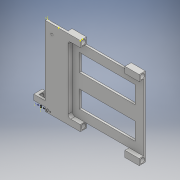
# Autodesk Inventor part: mtv_frontHolder(4_30)
Saved by Autodesk Inventor 2018 (Build 220112000, 112)
## iProperties
Created: 2019-04-30
Part Number: mtv_frontHolder(4_30)
Material: Generic
Document SubType Name: Modeling
Designer: Aditya Kendre
Density: 1 g/cm^3
Appearance: Default
Author: Aditya Kendre
## iProperties of the stored document mtv_frontHolder(4_30)_3DPrint.ipt
Created: 2019-04-30
Part Number: mtv_frontHolder(4_30)_3DPrint
Material: Generic
Document SubType Name: Modeling
Designer: Aditya Kendre
Density: 1 g/cm^3
Appearance: Default
Author: Aditya Kendre
Autodesk Inventor part; units mm, degrees
ref_plane "YZ Plane" through (0, 0, 0) normal (1, 0, 0) x (0, 1, 0)
ref_plane "XZ Plane" through (0, 0, 0) normal (0, 1, 0) x (-1, 0, 0)
ref_plane "XY Plane" through (0, 0, 0) normal (0, 0, 1) x (1, 0, 0)
sketch "Sketch1" plane through (0, 0, 0) normal (1, 0, 0) x (0, 1, 0)
  line L0 (0, 0) -> (8.763, 0)
  line L1 (8.763, 0) -> (8.763, -5.5118)
  line L2 (8.763, -5.5118) -> (0, -5.5118)
  line L3 (0, -5.5118) -> (0, 0)
  line L4 (1.5875, -3.9243) -> (7.1755, -3.9243)
  line L5 (7.1755, -3.9243) -> (7.1755, -1.5875)
  line L6 (7.1755, -1.5875) -> (1.5875, -1.5875)
  line L7 (1.5875, -1.5875) -> (1.5875, -3.9243)
  line L8 (1.5875, -3.9243) -> (7.1755, -1.5875) construction
  line L9 (7.1755, -3.9243) -> (1.5875, -1.5875) construction
  line L10 (0, -105.512) -> (8.763, -105.512)
  line L11 (8.763, -105.512) -> (8.763, -111.0238)
  line L12 (8.763, -111.0238) -> (0, -111.0238)
  line L13 (0, -111.0238) -> (0, -105.512)
  line L14 (1.5875, -109.4363) -> (7.1755, -109.4363)
  line L15 (7.1755, -109.4363) -> (7.1755, -107.0995)
  line L16 (7.1755, -107.0995) -> (1.5875, -107.0995)
  line L17 (1.5875, -107.0995) -> (1.5875, -109.4363)
  line L18 (1.5875, -109.4363) -> (7.1755, -107.0995) construction
  line L19 (7.1755, -109.4363) -> (1.5875, -107.0995) construction
  point P0 (4.3815, -2.7559)
  point P1 (4.3815, -108.2679)
  dimension "d0" = 8.763
  dimension "d1" = 5.5118
  dimension "d2" = 5.588
  dimension "d3" = 2.3368
  dimension "d4" = 8.763
  dimension "d5" = 5.5118
  dimension "d6" = 5.588
  dimension "d7" = 2.3368
  constraints: 40 end point, 8 parallel, 4 horizontal, 4 midpoint, 4 perpendicular, 1 point on line
  measures "d0" distance of L1.end L2.end
  measures "d1" distance of L0.end L1.end
  measures "d2" distance of L6.end L5.end
  measures "d3" distance of L5.end L4.end
  measures "d4" distance of L11.end L12.end
  measures "d5" distance of L10.end L11.end
  measures "d6" distance of L16.end L15.end
  measures "d7" distance of L15.end L14.end
extrude "Extrusion1" add sketch "Sketch1" against normal blind 30
sketch "Sketch2" plane through (-30, 0, 0) normal (-1, 0, 0) x (0, 0, 1)
  line L0 (0, 0) -> (0, 8.763) projected
  line L1 (-111.0238, 0) -> (0, 0)
  line L2 (0, 0) -> (0, 8.763)
  line L3 (0, 8.763) -> (-111.0238, 8.763)
  line L4 (-111.0238, 8.763) -> (-111.0238, 0)
  constraints: 8 end point, 2 parallel, 1 horizontal, 1 perpendicular
extrude "Extrusion2" add sketch "Sketch2" along normal blind 0.25
fillet "Fillet1" radius 5 2 edges at (-30, 4.3815, -5.5118) (-30, 4.3815, -105.512)
sketch "Sketch3" plane through (-30.25, 0, 0) normal (-1, 0, 0) x (0, 0, 1)
  point P0 (0, 0)
sketch "Sketch4" plane through (-30.25, 0, 0) normal (-1, 0, 0) x (0, 0, 1)
  line L0 (-111.0238, 8.763) -> (-111.0238, 0) projected
  line L1 (0, 0) -> (-111.0238, 0)
  line L2 (-111.0238, 0) -> (-111.0238, 3)
  line L3 (-111.0238, 3) -> (0, 3)
  line L4 (0, 3) -> (0, 0)
  dimension "d13" = 3
  constraints: 8 end point, 2 parallel, 1 horizontal, 1 perpendicular, 1 point on line
  measures "d13" distance of L1.end L2.end
extrude "Extrusion3" add sketch "Sketch4" along normal blind 18.97
sketch "Sketch5" plane through (-30.25, 3, 0) normal (0, 1, 0) x (1, 0, 0)
  line L0 (0, 0) -> (0, 111.0238) construction
  line L1 (0, 0) -> (-9.485, 0) construction
  line L2 (-9.485, 0) -> (-9.485, 6.985) construction
  line L3 (-9.485, 6.985) -> (0, 6.985) construction
  line L4 (0, 6.985) -> (0, 0) construction
  circle A0 centre (-9.485, 6.985) radius 1.5875
  point P0 (30.25, 0)
  dimension "d16" = 9.485
  dimension "d17" = 6.985
  dimension "d18" = 3.175
  constraints: 8 end point, 2 parallel, 1 centre point, 1 coincident, 1 horizontal, 1 perpendicular
  measures "d16" distance of L2.end L3.end
  measures "d17" distance of L1.end L2.end
  measures "d18" diameter of A0
extrude "Extrusion4" cut sketch "Sketch5" against normal blind 5
sketch "Sketch6" plane through (-30.25, 3, 0) normal (0, 1, 0) x (1, 0, 0)
  line L0 (30.25, 111.0238) -> (-18.97, 111.0238) construction
  line L1 (-28.07, 111.0238) -> (-28.07, 111.0238) construction
  line L2 (-28.07, 111.0238) -> (-28.07, 111.0238) construction
  line L3 (-28.07, 111.0238) -> (-28.07, 111.0238) construction
  line L4 (-28.07, 111.0238) -> (-28.07, 111.0238) construction
  line L5 (-28.07, 111.0238) -> (-28.07, 111.0238) construction
  line L6 (-28.07, 118.8238) -> (-28.07, 111.0238) construction
  line L7 (-28.07, 111.0238) -> (-37.17, 111.0238) construction
  line L8 (-37.17, 111.0238) -> (-37.17, 114.8988) construction
  line L9 (-28.07, 111.0238) -> (-28.07, 111.0238) construction
  line L10 (-28.07, 111.0238) -> (-28.07, 111.0238) construction
  line L11 (-28.07, 111.0238) -> (-28.07, 111.0238) construction
  line L12 (-28.07, 111.0238) -> (-28.07, 111.0238) construction
  line L13 (-28.07, 111.0238) -> (-28.07, 111.0238) construction
  line L14 (-28.07, 111.0238) -> (-28.07, 111.0238)
  line L15 (-28.07, 111.0238) -> (-28.07, 111.0238)
  line L16 (-28.07, 111.0238) -> (-28.07, 111.0238)
  line L17 (-28.07, 111.0238) -> (-28.07, 111.0238)
  point P0 (30.25, 0)
  dimension "d21" = 0
  dimension "d22" = 0
  dimension "d23" = 0
  dimension "d26" = 0
  dimension "d27" = 0
  constraints: 34 end point, 6 collinear, 4 horizontal, 4 perpendicular, 1 parallel, 1 point on line, 1 vertical
  measures "d21" distance of L3.end L2.end
  measures "d22" distance of L1.end L2.end
  measures "d23" distance of L2.end L5.end
  measures "d26" distance of L11.end L10.end
  measures "d27" distance of L9.start L10.end
sketch "Sketch7" plane through (-30.25, 3, 0) normal (0, 1, 0) x (1, 0, 0)
  line L0 (-18.97, 0) -> (-18.97, 111.0238) projected
  line L1 (-18.97, 111.0238) -> (-27.97, 111.0238)
  line L2 (-27.97, 111.0238) -> (-27.97, 103.2738)
  line L3 (-27.97, 103.2738) -> (-18.97, 103.2738)
  line L4 (-18.97, 103.2738) -> (-18.97, 111.0238)
  point P0 (30.25, 0)
  dimension "d28" = 9
  dimension "d29" = 7.75
  constraints: 8 end point, 2 parallel, 1 horizontal, 1 perpendicular
  measures "d28" distance of L3.end L2.end
  measures "d29" distance of L2.end L1.end
extrude "Extrusion5" add sketch "Sketch7" against normal blind 3
sketch "Sketch8" plane through (-30.25, 3, 0) normal (0, 1, 0) x (1, 0, 0)
  line L0 (-27.97, 111.0238) -> (-27.97, 103.2738) projected
  line L1 (-27.97, 111.0238) -> (-31.97, 111.0238)
  line L2 (-31.97, 111.0238) -> (-31.97, 103.2738)
  line L3 (-31.97, 103.2738) -> (-27.97, 103.2738)
  line L4 (-27.97, 103.2738) -> (-27.97, 111.0238)
  point P0 (30.25, 0)
  dimension "d32" = 4
  constraints: 8 end point, 2 parallel, 1 horizontal, 1 perpendicular
  measures "d32" distance of L3.end L2.end
extrude "Extrusion6" add sketch "Sketch8" along normal blind 8 and the other way blind 3
sketch "Sketch9" plane through (0, 0, -5.5118) normal (0, -1, 0) x (1, 0, 0)
  point P0 (0, 5.5118)
sketch "Sketch10" plane through (-62.22, 0, -103.2738) normal (-1, 0, 0) x (0, 0, 1)
  line L0 (-7.75, 0) -> (-2.2382, 0) construction
  line L1 (0, 3) -> (0, 11) construction
  line L2 (-7.75, 0) -> (0, 0) construction
  line L3 (0, 0) -> (0, 3) construction
  line L4 (0, 3) -> (-7.75, 3) construction
  line L5 (-7.75, 3) -> (-7.75, 0) construction
  line L6 (103.2738, 3) -> (0, 3) construction
  line L7 (-7.75, 8.763) -> (-7.75, 3) construction
  line L8 (0, 3) -> (-7.75, 3) construction
  line L9 (-7.75, 3) -> (-7.75, 6.875) construction
  line L10 (-7.75, 6.875) -> (0, 6.875) construction
  line L11 (0, 6.875) -> (0, 3) construction
  circle A0 centre (-3.875, 6.875) radius 3.1
  point P0 (103.2738, 0)
  dimension "d37" = 3.875
  dimension "d38" = 6.2
  constraints: 16 end point, 4 parallel, 2 horizontal, 2 perpendicular, 1 centre point, 1 midpoint, 1 point on line
  measures "d37" distance of L8.end L9.end
  measures "d38" diameter of A0
extrude "Extrusion7" cut sketch "Sketch10" against normal blind 5
sketch "Sketch11" plane through (0, 8.763, 0) normal (0, 1, 0) x (1, 0, 0)
  line L0 (-30.25, 111.0238) -> (-30.25, 0) projected
  line L1 (0, 0) -> (-30.25, 0) projected
  line L2 (-30.25, 111.0238) -> (-20.25, 111.0238)
  line L3 (-20.25, 111.0238) -> (-20.25, 0)
  line L4 (-20.25, 0) -> (-30.25, 0)
  line L5 (-30.25, 0) -> (-30.25, 111.0238)
  dimension "d41" = 10
  constraints: 8 end point, 2 parallel, 1 horizontal, 1 perpendicular, 1 point on line
  measures "d41" distance of L3.end L4.end
extrude "Extrusion8" cut sketch "Sketch11" against normal blind 10
sketch "Sketch12" plane through (-30.25, 0, 0) normal (1, 0, 0) x (0, 0, -1)
  line L0 (111.0238, 3) -> (111.0238, 0) projected
  line L1 (0, 0) -> (111.0238, 0)
  line L2 (111.0238, 0) -> (111.0238, 3)
  line L3 (111.0238, 3) -> (0, 3)
  line L4 (0, 3) -> (0, 0)
  constraints: 8 end point, 2 parallel, 1 horizontal, 1 perpendicular
extrude "Extrusion9" add sketch "Sketch12" along normal blind 13
sketch "Sketch13" plane through (0, 8.763, 0) normal (0, 1, 0) x (1, 0, 0)
  line L0 (-20.25, 5.5118) -> (-20.25, 0) projected
  line L1 (-62.22, 111.0238) -> (0, 111.0238) projected
  line L2 (-20.25, 0) -> (-17.25, 0)
  line L3 (-17.25, 0) -> (-17.25, 111.0238)
  line L4 (-17.25, 111.0238) -> (-20.25, 111.0238)
  line L5 (-20.25, 111.0238) -> (-20.25, 0)
  point P0 (0, 0)
  dimension "d46" = 3
  constraints: 8 end point, 2 parallel, 1 horizontal, 1 perpendicular, 1 point on line
  measures "d46" distance of L4.end L3.end
extrude "Extrusion10" add sketch "Sketch13" against normal blind 8.75
sketch "Sketch14" plane through (-49.22, 3, 0) normal (0, 1, 0) x (1, 0, 0)
  line L0 (-9, 111.0238) -> (28.97, 111.0238) construction
  line L1 (0, 0) -> (0, 0) construction
  line L2 (0, 0) -> (0, 111.0238) construction
  line L3 (0, 111.0238) -> (0, 111.0238) construction
  line L4 (0, 111.0238) -> (0, 0) construction
  point P0 (49.22, 0)
  dimension "d49" = 0
  constraints: 8 end point, 2 equal length, 1 horizontal, 1 perpendicular, 1 point on line
  measures "d49" distance of L3.end L2.end
sketch "Sketch15" plane through (-49.22, 3, 0) normal (0, 1, 0) x (1, 0, 0)
  line L0 (0, 107.1488) -> (28.97, 107.1488) construction
  line L1 (28.97, 111.0238) -> (28.97, 0) construction
  point P0 (49.22, 0)
  constraints: 2 end point, 1 horizontal, 1 point on line
sketch "Sketch16" plane through (-20.25, 8.763, -111.0238) normal (-1, 0, 0) x (0, 0, 1)
  line L0 (0, 0) -> (111.0238, 0) construction
  line L1 (0, 0) -> (7.7501, 0) construction
  line L2 (0, -5.763) -> (111.0238, -5.763) construction
  line L3 (0, 0) -> (7.7501, 0) construction
  line L4 (7.7501, 0) -> (7.7501, -5.763) construction
  line L5 (7.7501, -5.763) -> (0, -5.763) construction
  line L6 (0, -5.763) -> (0, 0) construction
  line L7 (0, -5.763) -> (4.375, -5.763) construction
  line L8 (4.375, -5.763) -> (4.375, -1.388) construction
  line L9 (4.375, -1.388) -> (0, -1.388) construction
  line L10 (0, -1.388) -> (0, -5.763) construction
  circle A0 centre (4.375, -1.388) radius 1.5
  point P0 (111.0238, -8.763)
  dimension "d52" = 4.375
  dimension "d53" = 4.375
  dimension "d54" = 3
  constraints: 18 end point, 4 parallel, 2 horizontal, 2 perpendicular, 2 point on line, 1 centre point, 1 coincident
  measures "d52" distance of L9.end L8.end
  measures "d53" distance of L8.end L7.end
  measures "d54" diameter of A0
extrude "Extrusion11" add sketch "Sketch16" along normal blind 2
sketch "Sketch17" plane through (-49.22, 3, 0) normal (0, 1, 0) x (1, 0, 0)
  circle A0 centre (9.485, 6.985) radius 1.5875 construction
  line L0 (0, 0) -> (0, 103.2738) construction
  line L1 (9.485, 6.985) -> (0, 6.985) construction
  line L2 (0, 6.985) -> (0, 0) construction
  line L3 (0, 0) -> (9.485, 0) construction
  line L4 (9.485, 0) -> (9.485, 6.985) construction
  line L5 (31.97, 5.5118) -> (31.97, 105.512) construction
  line L6 (31.97, 5.5118) -> (0, 5.5118) construction
  line L7 (0, 5.5118) -> (0, 12.4968) construction
  line L8 (0, 12.4968) -> (31.97, 12.4968) construction
  line L9 (31.97, 12.4968) -> (31.97, 5.5118) construction
  circle A1 centre (9.485, 12.4968) radius 1.5
  circle A2 centre (9.485, 6.985) radius 1.4732
  circle A3 centre (9.485, 6.985) radius 2.1184
  point P0 (49.22, 0)
  dimension "d57" = 9.485
  dimension "d58" = 6.985
  dimension "d59" = 6.985
  dimension "d60" = 3
  constraints: 16 end point, 4 parallel, 3 centre point, 3 coincident, 2 horizontal, 2 perpendicular, 2 point on line
  measures "d57" distance of L0.start L3.end
  measures "d58" distance of L0.start L1.end
  measures "d59" distance of L6.end L7.end
  measures "d60" diameter of A1
extrude "Extrusion12" cut sketch "Sketch17" against normal blind 3 contours A1
sketch "Sketch18" plane through (-49.22, 3, 0) normal (0, 1, 0) x (1, 0, 0)
  circle A0 centre (9.485, 6.985) radius 1.5875 projected
  circle A1 centre (9.485, 6.985) radius 2.2024
  point P0 (49.22, 0)
  constraints: 1 centre point, 1 coincident
extrude "Extrusion13" add sketch "Sketch18" against normal blind 3 contours A0 | A1
sketch "Sketch19" plane through (-49.22, 3, 0) normal (0, 1, 0) x (1, 0, 0)
  line L0 (49.22, 5.5118) -> (31.97, 5.5118) construction
  line L1 (31.97, 5.5118) -> (0, 5.5118) construction
  line L2 (31.97, 105.5118) -> (31.97, 5.5118) construction
  line L3 (0, 103.2738) -> (0, 0) construction
  line L4 (0, 103.2738) -> (-13.792, 103.2738) construction
  line L5 (-13.792, 103.2738) -> (-13.792, 112.9328) construction
  line L6 (-13.792, 112.9328) -> (0, 112.9328) construction
  line L7 (0, 112.9328) -> (0, 103.2738) construction
  line L8 (-9, 103.2738) -> (0, 103.2738) projected
  line L9 (0, 103.2738) -> (-14.6847, 103.2738)
  line L10 (-14.6847, 103.2738) -> (-14.6847, 119.5752)
  line L11 (-14.6847, 119.5752) -> (0, 119.5752)
  line L12 (0, 119.5752) -> (0, 103.2738)
  point P0 (49.22, 0)
  constraints: 20 end point, 4 parallel, 3 horizontal, 2 perpendicular
extrude "Extrusion14" cut sketch "Sketch19" along normal mid plane 30
sketch "Sketch20" plane through (-49.22, 3, 0) normal (0, 1, 0) x (1, 0, 0)
  line L0 (31.97, 5.5118) -> (31.97, 105.512) construction
  line L1 (0, 0) -> (0, 111.0238) construction
  line L2 (31.97, 5.5118) -> (0, 5.5118) construction
  line L3 (0, 5.5118) -> (0, 105.5118) construction
  line L4 (0, 105.5118) -> (31.97, 105.5118) construction
  line L5 (31.97, 105.5118) -> (31.97, 5.5118) construction
  line L6 (0, 105.5118) -> (-12.042, 105.5118)
  line L7 (-12.042, 105.5118) -> (-12.042, 97.7618)
  line L8 (-12.042, 97.7618) -> (0, 97.7618)
  line L9 (0, 97.7618) -> (0, 105.5118)
  point P0 (49.22, 0)
  dimension "d68" = 100
  dimension "d69" = 12.042
  dimension "d70" = 7.75
  constraints: 16 end point, 4 parallel, 2 horizontal, 2 perpendicular, 1 point on line
  measures "d68" distance of L2.end L3.end
  measures "d69" distance of L8.end L7.end
  measures "d70" distance of L7.end L6.end
extrude "Extrusion15" add sketch "Sketch20" against normal blind 3
sketch "Sketch21" plane through (-49.22, 3, 0) normal (0, 1, 0) x (1, 0, 0)
  line L0 (-12.042, 97.7618) -> (0, 97.7618) projected
  line L1 (-12.042, 97.7618) -> (-16.042, 97.7618)
  line L2 (-16.042, 97.7618) -> (-16.042, 105.5118)
  line L3 (-16.042, 105.5118) -> (-12.042, 105.5118)
  line L4 (-12.042, 105.5118) -> (-12.042, 97.7618)
  point P0 (49.22, 0)
  dimension "d73" = 4
  constraints: 8 end point, 2 parallel, 1 horizontal, 1 perpendicular
  measures "d73" distance of L2.end L3.end
extrude "Extrusion16" add sketch "Sketch21" along normal blind 9 and the other way blind 3
sketch "Sketch22" plane through (-65.262, 0, -97.7618) normal (-1, 0, 0) x (0, 0, 1)
  line L0 (-13.262, 3) -> (97.7618, 3) construction
  line L1 (0, 3) -> (-7.75, 3) construction
  line L2 (-7.75, 0) -> (-7.75, 3) construction
  line L3 (-7.75, 3) -> (-3.875, 3) construction
  line L4 (-3.875, 3) -> (-3.875, 6.875) construction
  line L5 (-3.875, 6.875) -> (-7.75, 6.875) construction
  line L6 (-7.75, 6.875) -> (-7.75, 3) construction
  circle A0 centre (-3.875, 6.875) radius 3.1
  point P0 (97.7618, 0)
  dimension "d78" = 7.75
  dimension "d79" = 3.875
  dimension "d80" = 3.875
  dimension "d81" = 6.2
  constraints: 10 end point, 2 parallel, 2 point on line, 1 centre point, 1 coincident, 1 horizontal, 1 perpendicular
  measures "d78" distance of L1.start L1.end
  measures "d79" distance of L5.end L4.end
  measures "d80" distance of L4.end L3.end
  measures "d81" diameter of A0
extrude "Extrusion17" cut sketch "Sketch22" against normal blind 4
sketch "Sketch23" plane through (-49.22, 3, 0) normal (0, 1, 0) x (1, 0, 0)
  point P0 (49.22, 0)
sketch "Sketch24" plane through (-20.25, 3, -111.0238) normal (-1, 0, 0) x (0, 0, 1)
  line L0 (0, 5.763) -> (3.8063, 5.763) construction
  line L1 (0, 0) -> (111.0238, 0) construction
  line L2 (0, 5.763) -> (5.512, 5.763) construction
  line L3 (5.512, 5.763) -> (5.512, 0) construction
  line L4 (5.512, 0) -> (0, 0) construction
  line L5 (0, 0) -> (0, 5.763) construction
  line L6 (5.512, 0) -> (9.887, 0) construction
  line L7 (9.887, 0) -> (9.887, 4.375) construction
  line L8 (9.887, 4.375) -> (5.512, 4.375) construction
  line L9 (5.512, 4.375) -> (5.512, 0) construction
  circle A0 centre (9.887, 4.375) radius 1.5
  point P0 (111.0238, -3)
  dimension "d84" = 5.512
  dimension "d85" = 4.375
  dimension "d86" = 4.375
  dimension "d87" = 3
  constraints: 16 end point, 4 parallel, 2 horizontal, 2 perpendicular, 1 centre point, 1 coincident, 1 point on line
  measures "d84" distance of L3.end L4.end
  measures "d85" distance of L8.end L7.end
  measures "d86" distance of L7.end L6.end
  measures "d87" diameter of A0
extrude "Extrusion18" add sketch "Sketch24" along normal blind 3
sketch "Sketch25" plane through (-22.25, 7.375, -106.6488) normal (-1, 0, 0) x (0, 0, 1)
  circle A0 centre (0, 0) radius 1.5
  point P0 (106.6488, -7.375)
  constraints: 1 centre point
extrude "Extrusion19" cut sketch "Sketch25" against normal blind 2
sketch "Sketch26" plane through (0, 0, 0) normal (1, 0, 0) x (0, 0, -1)
  line L0 (0, 0) -> (0, 8.763) projected
  line L1 (0, 8.763) -> (8.763, 8.763)
  line L2 (8.763, 8.763) -> (8.763, 0)
  line L3 (8.763, 0) -> (0, 0)
  line L4 (0, 0) -> (0, 8.763)
  line L5 (105.512, 8.763) -> (111.0238, 8.763) projected
  line L6 (5.5118, 0) -> (105.512, 0) projected
  line L7 (111.0238, 8.763) -> (102.2608, 8.763)
  line L8 (102.2608, 8.763) -> (102.2608, 0)
  line L9 (102.2608, 0) -> (111.0238, 0)
  line L10 (111.0238, 0) -> (111.0238, 8.763)
  dimension "d92" = 8.763
  dimension "d93" = 8.763
  constraints: 16 end point, 4 parallel, 2 horizontal, 2 perpendicular, 1 point on line
  measures "d92" distance of L2.end L3.end
  measures "d93" distance of L9.end L8.end
extrude "Extrusion20" add sketch "Sketch26" against normal blind 20.25
sketch "Sketch27" plane through (-49.22, 3, 0) normal (0, 1, 0) x (1, 0, 0)
  point P0 (49.22, 0)
sketch "Sketch28" plane through (0, 0, 0) normal (1, 0, 0) x (0, 0, -1)
  line L0 (0, 8.763) -> (8.763, 8.763) construction
  line L1 (0, 8.763) -> (8.763, 0) construction
  line L2 (8.763, 0) -> (8.763, 8.763) construction
  line L3 (97.7618, 0) -> (0, 0) construction
  line L4 (8.763, 8.763) -> (0, 0) construction
  line L5 (111.0238, 8.763) -> (102.2608, 8.763) construction
  line L6 (111.0238, 8.763) -> (111.0238, 0) construction
  line L7 (102.2608, 8.763) -> (111.0238, 0) construction
  line L8 (111.0238, 0) -> (111.0238, 8.763) construction
  line L9 (111.0238, 8.763) -> (102.2608, 0) construction
  circle A0 centre (106.6423, 4.3815) radius 3.25
  circle A1 centre (4.3815, 4.3815) radius 3.25
  dimension "d96" = 6.5
  dimension "d97" = 6.5
  constraints: 12 end point, 2 centre point, 2 midpoint, 2 perpendicular, 1 collinear, 1 vertical
  measures "d96" diameter of A0
  measures "d97" diameter of A1
extrude "Extrusion21" cut sketch "Sketch28" against normal blind 17.25
fillet "Fillet2" radius 4 2 edges at (-17.25, 4.3815, -8.763) (-17.25, 4.3815, -102.2608)
sketch "Sketch29" plane through (-17.25, 0, 0) normal (1, 0, 0) x (0, 0, -1)
  line L0 (8.763, 0) -> (8.763, 8.763) projected
  line L1 (102.2608, 0) -> (102.2608, 8.763) projected
  line L2 (8.763, 8.763) -> (102.2608, 8.763)
  line L3 (102.2608, 8.763) -> (102.2608, 6.013)
  line L4 (102.2608, 6.013) -> (8.763, 6.013)
  line L5 (8.763, 6.013) -> (8.763, 8.763)
  point P0 (0, 0)
  dimension "d101" = 2.75
  constraints: 8 end point, 2 parallel, 1 horizontal, 1 perpendicular, 1 point on line
  measures "d101" distance of L2.end L3.end
extrude "Extrusion22" add sketch "Sketch29" along normal blind 100
sketch "Sketch30" plane through (-20.25, 8.763, -111.0238) normal (0, 1, 0) x (1, 0, 0)
  line L0 (103, -102.2608) -> (103, -8.763) construction
  line L1 (103, -102.2608) -> (3, -102.2608) construction
  line L2 (3, -102.2608) -> (3, -8.763) construction
  line L3 (3, -8.763) -> (103, -8.763) construction
  line L4 (103, -8.763) -> (103, -102.2608) construction
  line L5 (3, -98.2608) -> (3, -12.763) construction
  line L6 (3, -55.5119) -> (103, -55.5119) construction
  line L7 (3, -55.5119) -> (101.425, -55.5119) construction
  line L8 (101.425, -55.5119) -> (101.425, -99.9619) construction
  line L9 (101.425, -99.9619) -> (3, -99.9619) construction
  line L10 (3, -99.9619) -> (3, -55.5119) construction
  line L11 (3, -55.5119) -> (101.425, -55.5119) construction
  line L12 (101.425, -55.5119) -> (101.425, -11.0619) construction
  line L13 (101.425, -11.0619) -> (3, -11.0619) construction
  line L14 (3, -11.0619) -> (3, -55.5119) construction
  line L15 (101.425, -55.5119) -> (91.425, -55.5119) construction
  line L16 (91.425, -55.5119) -> (91.425, -11.0619) construction
  line L17 (91.425, -11.0619) -> (91.425, -21.0619) construction
  line L18 (91.425, -21.0619) -> (3, -21.0619) construction
  line L19 (13, -21.0619) -> (13, -99.9619) construction
  line L20 (13, -99.9619) -> (13, -89.9619) construction
  line L21 (13, -89.9619) -> (101.425, -89.9619) construction
  line L22 (91.425, -55.5119) -> (91.425, -89.9619) construction
  line L23 (13, -89.9619) -> (91.425, -89.9619)
  line L24 (91.425, -89.9619) -> (91.425, -21.0619)
  line L25 (91.425, -21.0619) -> (13, -21.0619)
  line L26 (13, -21.0619) -> (13, -89.9619)
  point P0 (20.25, -111.0238)
  dimension "d104" = 100
  dimension "d105" = 98.425
  dimension "d106" = 44.45
  dimension "d107" = 44.45
  dimension "d108" = 10
  dimension "d109" = 10
  dimension "d110" = 10
  constraints: 50 end point, 10 point on line, 8 parallel, 8 perpendicular, 4 horizontal, 2 midpoint
  measures "d104" distance of L2.end L3.end
  measures "d105" distance of L8.end L9.end
  measures "d106" distance of L7.end L8.end
  measures "d107" distance of L12.end L11.end
  measures "d108" distance of L11.end L15.end
  measures "d109" distance of L16.end L17.end
  measures "d110" distance of L19.end L20.end
extrude "Extrusion23" cut sketch "Sketch30" against normal blind 5
sketch "Sketch31" plane through (-20.25, 8.763, -111.0238) normal (0, 1, 0) x (1, 0, 0)
  line L0 (13, -89.9619) -> (13, -21.0619) construction
  line L1 (13, -55.5119) -> (91.425, -55.5119) construction
  line L2 (91.425, -89.9619) -> (91.425, -21.0619) construction
  line L3 (91.425, -45.5119) -> (13, -45.5119)
  line L4 (13, -45.5119) -> (13, -65.5119)
  line L5 (13, -65.5119) -> (91.425, -65.5119)
  line L6 (91.425, -65.5119) -> (91.425, -45.5119)
  line L7 (91.425, -45.5119) -> (13, -65.5119) construction
  line L8 (13, -45.5119) -> (91.425, -65.5119) construction
  point P0 (20.25, -111.0238)
  point P1 (52.2125, -55.5119)
  dimension "d113" = 20
  constraints: 14 end point, 5 midpoint, 2 parallel, 1 horizontal, 1 perpendicular, 1 point on line
  measures "d113" distance of L4.end L3.end
extrude "Extrusion24" add sketch "Sketch31" against normal blind 2.75
sketch "Sketch32" plane through (82.75, 0, 0) normal (1, 0, 0) x (0, 0, -1)
  line L0 (8.763, 8.763) -> (8.763, 6.013) projected
  line L1 (0, 0) -> (8.763, 0) projected
  line L2 (8.763, 8.763) -> (0, 8.763)
  line L3 (0, 8.763) -> (0, 0)
  line L4 (0, 0) -> (8.763, 0)
  line L5 (8.763, 0) -> (8.763, 8.763)
  line L6 (111.0238, 8.763) -> (111.0238, 0) projected
  line L7 (102.2608, 8.763) -> (111.0238, 8.763)
  line L8 (111.0238, 8.763) -> (111.0238, 0)
  line L9 (111.0238, 0) -> (102.2608, 0)
  line L10 (102.2608, 0) -> (102.2608, 8.763)
  circle A0 centre (106.6423, 4.3815) radius 3.25
  circle A1 centre (4.3815, 4.3815) radius 3.25 projected
  circle A2 centre (4.3815, 4.3815) radius 3.25
  constraints: 16 end point, 4 parallel, 2 centre point, 2 horizontal, 2 perpendicular, 1 coincident
extrude "Extrusion25" add sketch "Sketch32" against normal blind 20
body "Solid1"
